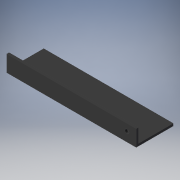
# Autodesk Inventor part: Switch-Panel-Divider
Saved by Autodesk Inventor 2018 (Build 220112000, 112)
## iProperties
Created: 2018-08-13
Part Number: Switch-Panel-Divider
Material: Generic
Document SubType Name: Modeling
Designer: bbramman
Density: 1 g/cm^3
Appearance: Default
Author: bbramman
Autodesk Inventor part; units mm, degrees
ref_plane "YZ Plane" through (0, 0, 0) normal (1, 0, 0) x (0, 1, 0)
ref_plane "XZ Plane" through (0, 0, 0) normal (0, 1, 0) x (-1, 0, 0)
ref_plane "XY Plane" through (0, 0, 0) normal (0, 0, 1) x (1, 0, 0)
sketch "Sketch1" plane through (0, 0, 0) normal (0, 1, 0) x (-1, 0, 0)
  line L0 (-44.45, 12.7) -> (44.45, 12.7)
  line L1 (44.45, 12.7) -> (44.45, -12.7)
  line L2 (44.45, -12.7) -> (-44.45, -12.7)
  line L3 (-44.45, -12.7) -> (-44.45, 12.7)
  line L4 (-44.45, 12.7) -> (44.45, -12.7) construction
  line L5 (44.45, 12.7) -> (-44.45, -12.7) construction
  point P0 (0, 0)
  dimension "d0" = 88.9
  dimension "d1" = 25.4
  constraints: 12 end point, 2 midpoint, 2 parallel, 1 horizontal, 1 perpendicular
  measures "d0" distance of L1.end L2.end
  measures "d1" distance of L0.end L1.end
extrude "Extrusion1" add sketch "Sketch1" along normal blind 1.5875
sketch "Sketch2" plane through (0, 1.5875, 0) normal (0, 1, 0) x (1, 0, 0)
  line L0 (-44.45, -12.7) -> (44.45, -12.7) projected
  line L1 (-44.45, -12.7) -> (-44.45, -11.1125)
  line L2 (-44.45, 12.7) -> (-44.45, -12.7) projected
  line L3 (-44.45, -11.1125) -> (44.45, -11.1125)
  line L4 (44.45, -11.1125) -> (44.45, -12.7)
  line L5 (44.45, -12.7) -> (-44.45, -12.7)
  line L6 (-44.45, -12.7) -> (-44.45, -11.1125)
  point P0 (0, 0)
  dimension "d4" = 1.5875
  constraints: 10 end point, 2 parallel, 1 horizontal, 1 perpendicular, 1 point on line
  measures "d4" distance of L0.start L1.end
extrude "Extrusion2" add sketch "Sketch2" along normal blind 9.525
sketch "Sketch3" plane through (44.45, 1.5875, 11.1125) normal (0, 0, -1) x (-1, 0, 0)
  line L0 (0, -1.5875) -> (0, 9.525) projected
  line L1 (0, 9.525) -> (6.35, 9.525)
  line L2 (88.9, 9.525) -> (0, 9.525) projected
  line L3 (88.9, 0) -> (0, 0) projected
  line L4 (88.9, 0) -> (88.9, 9.525) projected
  line L5 (0, 9.525) -> (88.9, 9.525) projected
  line L6 (0, 0) -> (0, 9.525) projected
  line L7 (0, 0) -> (88.9, 0) projected
  line L8 (6.35, 9.525) -> (6.35, 4.7625)
  circle A0 centre (6.35, 4.7625) radius 1.4351
  point P0 (44.45, -1.5875)
  dimension "d7" = 6.35
  dimension "d8" = 2.8702
  constraints: 4 end point, 1 centre point, 1 coincident, 1 perpendicular, 1 point on line
  measures "d7" distance of L0.end L1.end
  measures "d8" diameter of A0
extrude "Extrusion3" cut sketch "Sketch3" against normal through all contours A0
body "Solid1"
